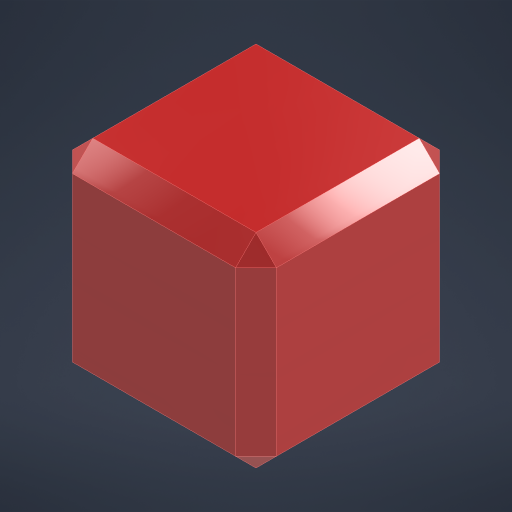
# Autodesk Inventor part: CUBE
Saved by Autodesk Inventor 2023 (Build 270158000, 158)
## iProperties
Created: 2023-03-04
Part Number: CUBE
Material: Generic
Document SubType Name: Modeling
Designer: Phoenix
Density: 1 g/cm^3
Appearance: Red
Author: Phoenix
Autodesk Inventor part; units mm, degrees
ref_plane "YZ Plane" through (0, 0, 0) normal (1, 0, 0) x (0, 1, 0)
ref_plane "XZ Plane" through (0, 0, 0) normal (0, 1, 0) x (-1, 0, 0)
ref_plane "XY Plane" through (0, 0, 0) normal (0, 0, 1) x (1, 0, 0)
sketch "Sketch1" plane through (0, 0, 0) normal (0, 1, 0) x (-1, 0, 0)
  line L0 (0, 0) -> (-50, 0)
  line L1 (-50, 0) -> (-50, 50)
  line L2 (-50, 50) -> (0, 50)
  line L3 (0, 50) -> (0, 0)
  dimension "d0" = 50
  dimension "d1" = 50
  constraints: 8 end point, 2 parallel, 1 horizontal, 1 perpendicular
  measures "d0" distance of L1.end L2.end
  measures "d1" distance of L0.end L1.end
extrude "Extrusion1" add sketch "Sketch1" along normal blind 50
chamfer "Chamfer1" distance 5 angle 45 12 edges at (25, 0, 50) (50, 0, 25) (25, 50, 0) (25, 0, 0) (0, 25, 0) (0, 50, 25) (0, 25, 50) (0, 0, 25) (25, 50, 50) (50, 25, 50) (50, 50, 25) (50, 25, 0)
body "Solid1"
